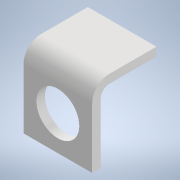
# Autodesk Inventor part: WheelMount No Motor
Saved by Autodesk Inventor 2022.2 (Build 262287000, 287)
## iProperties
Created: 2022-04-01
Part Number: WheelMount No Motor
Material: Generic
Document SubType Name: Sheet Metal
Designer: foriw
Density: 1 g/cm^3
Sheet Metal Rule: Default_mm
Appearance: Default
Author: foriw
Autodesk Inventor part; units mm, degrees
ref_plane "YZ Plane" through (0, 0, 0) normal (1, 0, 0) x (0, 1, 0)
ref_plane "XZ Plane" through (0, 0, 0) normal (0, 1, 0) x (-1, 0, 0)
ref_plane "XY Plane" through (0, 0, 0) normal (0, 0, 1) x (1, 0, 0)
sketch "Sketch1" plane through (0, 0, 0) normal (0, 1, 0) x (-1, 0, 0)
  line L0 (-8, 7.5) -> (8, 7.5)
  line L1 (8, 7.5) -> (8, -7.5)
  line L2 (8, -7.5) -> (-8, -7.5)
  line L3 (-8, -7.5) -> (-8, 7.5)
  line L4 (-8, 7.5) -> (8, -7.5) construction
  line L5 (8, 7.5) -> (-8, -7.5) construction
  point P0 (0, 0)
  dimension "d0" = 16
  dimension "d1" = 15
  constraints: 12 end point, 2 midpoint, 2 parallel, 1 horizontal, 1 perpendicular
  measures "d0" distance of L1.end L2.end
  measures "d1" distance of L0.end L1.end
extrude "Extrusion1" add sketch "Sketch1" against normal blind 2
sketch "Sketch2" plane through (-8, 0, 5.5) normal (0, 0, 1) x (1, 0, 0)
  line L0 (16, 0) -> (0, 0)
  line L1 (0, 0) -> (0, -18)
  line L2 (0, -18) -> (16, -18)
  line L3 (16, -18) -> (16, 0)
  constraints: 6 end point, 1 horizontal, 1 perpendicular, 1 vertical
edge flange "Flange1" height 18 angle 90 thickness 2 bend radius 2 thickness toward (0, 0, 1) relief tear relief width 2 relief depth 1 edges at (0, -2, 7.5) wall of the first edge with corners at (8, 0, 5.5) (-8, 0, 5.5) (-8, -18, 5.5) (8, -18, 5.5)
bend "Bend1"
corner "Corner1"
sketch "Sketch3" plane through (8, -18, 5.5) normal (0, 0, -1) x (-1, 0, 0)
  line L0 (16, 14) -> (0, 14) projected
  line L1 (0, 14) -> (0, 0) projected
  line L2 (0, 0) -> (16, 0) projected
  line L3 (16, 14) -> (16, 0) projected
  line L4 (16, 14) -> (0, 14) projected
  line L5 (16, 16) -> (16, 14) projected
  line L6 (0, 16) -> (16, 16) projected
  line L7 (0, 16) -> (0, 14) projected
  line L8 (0, 0) -> (16, 0) projected
  line L9 (8, 0) -> (8, 16) construction
  point P0 (8, 18)
  point P1 (8, 8)
  dimension "d15" = 8
  constraints: 3 midpoint, 2 end point
  measures "d15" distance from line of point (8, 8) L2
hole "Hole1" at (0, -10, 5.5) direction (0, 0, 1) diameter 10 end through all
equation "\"d21\" = Thickness"
equation "\"d4\" = Thickness"
equation "\"d5\" = BendReliefWidth"
equation "\"d6\" = BendReliefDepth"
equation "\"d7\" = MinimumRemnant"
equation "\"d8\" = TransitionRadius"
equation "\"d11\" = BendRadius"
equation "\"d12\" = CornerReliefSize"
equation "\"d13\" = GapSize"
equation "\"d14\" = JacobiRadiusSize"
equation "\"BendRadius\" = Thickness"
equation "\"BendReliefWidth\" = Thickness"
equation "\"BendReliefDepth\" = 0.5 * Thickness"
equation "\"CornerReliefSize\" = 4 * Thickness"
equation "\"MinimumRemnant\" = 2 * Thickness"
equation "\"TransitionRadius\" = BendRadius"
equation "\"JacobiRadiusSize\" = BendRadius"
equation "\"GapSize\" = Thickness"
equation "\"Thickness\" = 2"
body "Solid1"
